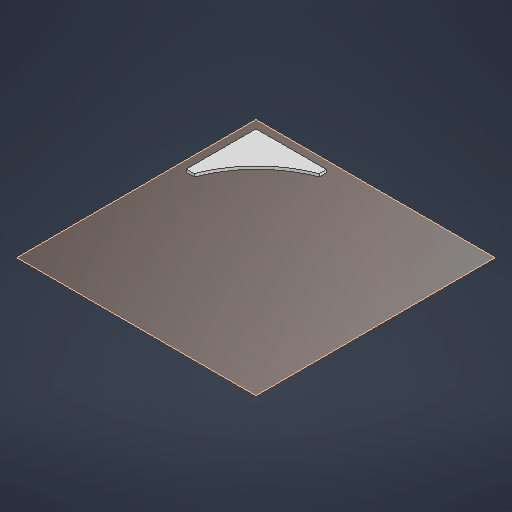
# Autodesk Inventor part: Roh
Saved by Autodesk Inventor 2026.2 (Build 302298000, 298)
## iProperties
Created: 2026-04-13
Part Number: Roh
Material: Všeobecné
Document SubType Name: Modeling
Designer: cerna
Density: 1 g/cm^3
Appearance: Výchozí
Author: cerna
Autodesk Inventor part; units mm, degrees
ref_plane "YZ Plane" through (0, 0, 0) normal (1, 0, 0) x (0, 1, 0)
ref_plane "XZ Plane" through (0, 0, 0) normal (0, 1, 0) x (-1, 0, 0)
ref_plane "XY Plane" through (0, 0, 0) normal (0, 0, 1) x (1, 0, 0)
ref_plane "Pracovní rovina1" through (0, 0, 0) normal (0, 0, 1) x (1, 0, 0)
sketch "Náčrt1" plane through (0, 0, 0) normal (0, 0, 1) x (1, 0, 0)
  line L0 (16.5, 77.5) -> (20.5568, 77.5) projected
  arc A0 (71, 129.8156) -> (20.5568, 77.5) centre (75.5, 75) ccw projected
  line L1 (71, 129.8156) -> (71, 145) projected
  line L2 (71, 145) -> (48.5742, 145) projected
  arc A1 (48.5742, 145) -> (5.5, 101.9258) centre (75.5, 75) ccw projected
  line L3 (5.5, 101.9258) -> (5.5, 48.0742) projected
  arc A2 (5.5, 48.0742) -> (48.5742, 5) centre (75.5, 75) ccw projected
  line L4 (48.5742, 5) -> (102.4258, 5) projected
  arc A3 (102.4258, 5) -> (145.5, 48.0742) centre (75.5, 75) ccw projected
  line L5 (145.5, 48.0742) -> (145.5, 101.9258) projected
  arc A4 (145.5, 101.9258) -> (102.4258, 145) centre (75.5, 75) ccw projected
  line L6 (102.4258, 145) -> (80, 145) projected
  line L7 (80, 145) -> (80, 129.8156) projected
  arc A5 (130.4181, 78) -> (80, 129.8156) centre (75.5, 75) ccw projected
  line L8 (130.4181, 78) -> (134.5, 78) projected
  line L9 (134.5, 78) -> (134.5, 72) projected
  line L10 (134.5, 72) -> (130.4181, 72) projected
  arc A6 (20.5568, 72.5) -> (130.4181, 72) centre (75.5, 75) ccw projected
  line L11 (20.5568, 72.5) -> (16.5, 72.5) projected
  line L12 (16.5, 72.5) -> (16.5, 77.5) projected
  line L13 (0, 150) -> (150, 150) projected
  line L14 (0, 0) -> (0, 150) projected
  line L15 (145, 5) -> (5, 5) projected
  line L16 (5, 5) -> (5, 72.5) projected
  line L17 (5, 72.5) -> (9, 72.5) projected
  line L18 (9, 77.5) -> (9, 72.5) projected
  line L19 (5, 77.5) -> (9, 77.5) projected
  line L20 (5, 77.5) -> (5, 145) projected
  line L21 (5, 145) -> (145, 145) projected
  line L22 (145, 145) -> (145, 77.5) projected
  line L23 (145, 77.5) -> (141, 77.5) projected
  line L24 (141, 72.5) -> (141, 77.5) projected
  line L25 (145, 72.5) -> (141, 72.5) projected
  line L26 (145, 72.5) -> (145, 5) projected
  line L27 (0, 0) -> (150, 0) projected
  line L28 (150, 0) -> (150, 150) projected
  line L29 (0, 150) -> (150, 150) projected
  line L30 (0, 0) -> (0, 150) projected
  line L31 (48.5742, 145) -> (5, 145)
  line L32 (48.5742, 145) -> (48.5742, 150)
  line L33 (48.5742, 150) -> (0, 150)
  line L34 (0, 150) -> (0, 101.9258)
  line L35 (5.5, 101.9258) -> (0, 101.9258)
  arc A7 (48.5742, 145) -> (5.5, 101.9258) centre (75.5, 75) ccw
  constraints: 10 end point, 3 perpendicular, 2 concentric, 2 point on circle, 2 point on line, 1 centre point, 1 collinear
extrude "Vysunutí1" add sketch "Náčrt1" along normal blind 2 contours A1 L35 L20 L21 | L21 L20 L35 L14 L13 L32
